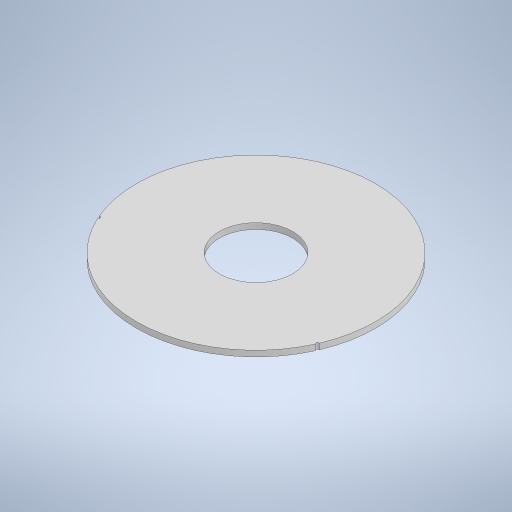
# Autodesk Inventor part: ДМФ 032 крышка Нос
Saved by Autodesk Inventor 2024.2 (Build 282272000, 272)
## iProperties
Created: 2024-04-23
Part Number: ДМФ 032 крышка Нос
Material: Generic
Document SubType Name: Sheet Metal
Designer: admin
Density: 1 g/cm^3
Appearance: Default
Stock Number: ДМФ 032 крышка Нос
Flat Pattern Width: 41 cm
Flat Pattern Length: 41 cm
Flat Pattern Area: 1681 cm^2
Sheet Metal Rule: Default
Sheet Metal Width: 410,000 mm
Sheet Metal Length: 410,000 mm
Sheet Metal Area: 168100,000 mm^2
Author: admin
Autodesk Inventor part; units mm, degrees
ref_plane "YZ Plane" through (0, 0, 0) normal (1, 0, 0) x (0, 1, 0)
ref_plane "XZ Plane" through (0, 0, 0) normal (0, 1, 0) x (-1, 0, 0)
ref_plane "XY Plane" through (0, 0, 0) normal (0, 0, 1) x (1, 0, 0)
sketch "Sketch1" plane through (0, 0, 0) normal (0, 0, 1) x (1, 0, 0)
  circle A0 centre (0, 0) radius 195 construction
  circle A1 centre (0, 0) radius 205
  circle A2 centre (0, 0) radius 63
  dimension "d0" = 390
  dimension "d4" = 126
  dimension "d13" = 10
  constraints: 3 centre point, 3 coincident
  measures "d0" diameter of A0
  measures "d4" diameter of A2
  measures "d13" radial gap between concentric circles of A1 A0
extrude "Extrusion1" add sketch "Sketch1" along normal blind 10
sketch "Sketch3" plane through (0, 0, 0) normal (0, 0, -1) x (-1, 0, 0)
  circle A0 centre (0, 0) radius 205 construction
  circle A1 centre (-187.6666, -82.5) radius 2.5
  circle A2 centre (187.6666, -82.5) radius 2.5
  line L0 (-187.6666, -82.5) -> (187.6666, -82.5) construction
  dimension "d14" = 5
  dimension "d15" = 82.5
  constraints: 2 centre point, 2 end point, 2 point on circle, 1 equal radius, 1 horizontal
  measures "d14" diameter of A1
  measures "d15" distance from line of L0 point (0, 0)
extrude "Extrusion3" cut sketch "Sketch3" against normal through all
equation "\"d0\" = Шпил_пласт_НОС_диам_центров"
equation "\"d4\" = Стенка_НОС_диам_илоотвод"
equation "\"d2\" = Thickness"
equation "\"BendReliefDepth\" = 0.5 * Thickness"
equation "\"Шпил_пласт_НОС_диам_центров\" = 390"
equation "\"Стенка_НОС_диам_илоотвод\" = 126"
equation "\"Thickness\" = 10"
body "Solid1"
